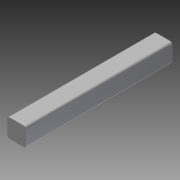
# Autodesk Inventor part: Vex Shaft P2
Saved by Autodesk Inventor 2014 SP1 (Build 180222100, 222)
## iProperties
Created: 2012-02-13
Part Number: Vex Shaft P2
Material: Steel
Document SubType Name: Modeling
Designer: Moses
Density: 7.85 g/cm^3
Mass: 2.04996 g
Surface Area: 3.31689 cm^2
Volume: 0.261142 cm^3
Appearance: Steel
Author: Moses
Autodesk Inventor part; units mm, degrees
ref_plane "YZ Plane" through (0, 0, 0) normal (1, 0, 0) x (0, 1, 0)
ref_plane "XZ Plane" through (0, 0, 0) normal (0, 1, 0) x (-1, 0, 0)
ref_plane "XY Plane" through (0, 0, 0) normal (0, 0, 1) x (1, 0, 0)
sketch "Sketch1" plane through (0, 0, 0) normal (0, 0, 1) x (1, 0, 0)
  line L0 (0, 0) -> (0, 3.2258)
  line L1 (0, 3.2258) -> (3.2258, 3.2258)
  line L2 (3.2258, 3.2258) -> (3.2258, 0)
  line L3 (3.2258, 0) -> (0, 0)
  dimension "d0" = 3.2258
  dimension "d1" = 3.2258
  constraints: 8 end point, 2 parallel, 1 perpendicular, 1 vertical
  measures "d0" distance of L0.start L0.end
  measures "d1" distance of L0.end L1.end
extrude "Extrusion1" add sketch "Sketch1" along normal blind 25.4
fillet "Fillet1" radius 0.381 4 edges at (3.2258, 3.2258, 12.7) (3.2258, 0, 12.7) (0, 3.2258, 12.7) (0, 0, 12.7)
ref_plane "Work Plane1" through (1.6129, 0.381, 25.4) normal (1, 0, 0) x (0, 0, -1)
ref_plane "Work Plane2" through (0.381, 1.6129, 25.4) normal (0, 1, 0) x (1, 0, 0)
body "Solid1"
